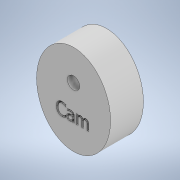
# Autodesk Inventor part: OVAAAAAL cam
Saved by Autodesk Inventor 2021 (Build 250183000, 183)
## iProperties
Created: 2021-04-14
Part Number: OVAAAAAL cam
Material: Generic
Document SubType Name: Modeling
Designer: Nabeel Azafer
Density: 1 g/cm^3
Appearance: Default
Author: Nabeel Azafer
Autodesk Inventor part; units mm, degrees
note: some values were not read from the file. Chosen so that the rebuilt part matches the saved one: direction of "Emboss1".
ref_plane "YZ Plane" through (0, 0, 0) normal (1, 0, 0) x (0, 1, 0)
ref_plane "XZ Plane" through (0, 0, 0) normal (0, 1, 0) x (-1, 0, 0)
ref_plane "XY Plane" through (0, 0, 0) normal (0, 0, 1) x (1, 0, 0)
sketch "Sketch1" plane through (0, 0, 0) normal (0, 0, 1) x (1, 0, 0)
  ellipse E0 centre (0, 0) end of major axis (0, 11) minor radius 9
  circle A0 centre (0, 3.5) radius 1.5
  dimension "d0" = 9
  dimension "d1" = 11
  dimension "d2" = 3
  dimension "d3" = 3.5
  constraints: 1 centre point, 1 coincident, 2 other
  measures "d2" diameter of A0
  measures "d3" distance of point (0, 0) A0.centre
extrude "Extrusion1" add sketch "Sketch1" along normal blind 8
sketch "Sketch2" plane through (0, 0, 8) normal (0, 0, 1) x (1, 0, 0)
  line L0 (-4.2953, -1.7977) -> (3.1049, -1.7977) construction
  line L1 (3.1049, -1.7977) -> (3.1049, -5.4978) construction
  line L2 (3.1049, -5.4978) -> (-4.2953, -5.4978) construction
  line L3 (-4.2953, -5.4978) -> (-4.2953, -1.7977) construction
  spline S0 degree 2 poles (-2.796, -4.9544) (-3.0924, -4.9544) (-3.5938, -4.7543) (-3.7766, -4.5542) knots 0 0 0 1 2 2 2
  spline S1 degree 2 poles (-3.7766, -4.5542) (-3.9594, -4.3566) (-4.1595, -3.7638) (-4.1595, -3.3785) knots 0 0 0 1 2 2 2
  spline S2 degree 2 poles (-4.1595, -3.3785) (-4.1595, -2.9956) (-3.9643, -2.4275) (-3.7791, -2.2176) knots 0 0 0 1 2 2 2
  spline S3 degree 2 poles (-3.7791, -2.2176) (-3.5963, -2.0126) (-3.0974, -1.7977) (-2.7886, -1.7977) knots 0 0 0 1 2 2 2
  spline S4 degree 2 poles (-2.7886, -1.7977) (-2.6355, -1.7977) (-2.3662, -1.8421) (-2.2526, -1.8767) knots 0 0 0 1 2 2 2
  spline S5 degree 2 poles (-2.2526, -1.8767) (-2.1538, -1.9088) (-1.9488, -2.0002) (-1.8475, -2.0546) knots 0 0 0 1 2 2 2
  line L4 (-1.8475, -2.0546) -> (-1.8475, -2.5436)
  line L5 (-1.8475, -2.5436) -> (-1.8796, -2.5436)
  spline S6 degree 2 poles (-1.8796, -2.5436) (-1.934, -2.4942) (-2.1019, -2.3559) (-2.223, -2.2892) knots 0 0 0 1 2 2 2
  spline S7 degree 2 poles (-2.223, -2.2892) (-2.3391, -2.225) (-2.6132, -2.1435) (-2.7911, -2.1435) knots 0 0 0 1 2 2 2
  spline S8 degree 2 poles (-2.7911, -2.1435) (-2.9862, -2.1435) (-3.3345, -2.304) (-3.4654, -2.4572) knots 0 0 0 1 2 2 2
  spline S9 degree 2 poles (-3.4654, -2.4572) (-3.5938, -2.6128) (-3.7371, -3.0846) (-3.7371, -3.3785) knots 0 0 0 1 2 2 2
  spline S10 degree 2 poles (-3.7371, -3.3785) (-3.7371, -3.6922) (-3.5864, -4.1442) (-3.4555, -4.2998) knots 0 0 0 1 2 2 2
  spline S11 degree 2 poles (-3.4555, -4.2998) (-3.3271, -4.4505) (-2.9837, -4.6036) (-2.7911, -4.6036) knots 0 0 0 1 2 2 2
  spline S12 degree 2 poles (-2.7911, -4.6036) (-2.6157, -4.6036) (-2.3168, -4.5172) (-2.2007, -4.4529) knots 0 0 0 1 2 2 2
  spline S13 degree 2 poles (-2.2007, -4.4529) (-2.0896, -4.3887) (-1.9241, -4.2553) (-1.8772, -4.2084) knots 0 0 0 1 2 2 2
  line L6 (-1.8772, -4.2084) -> (-1.8475, -4.2084)
  line L7 (-1.8475, -4.2084) -> (-1.8475, -4.6925)
  spline S14 degree 2 poles (-1.8475, -4.6925) (-1.9488, -4.7395) (-2.1266, -4.8259) (-2.2526, -4.8654) knots 0 0 0 1 2 2 2
  spline S15 degree 2 poles (-2.2526, -4.8654) (-2.386, -4.9099) (-2.6132, -4.9544) (-2.796, -4.9544) knots 0 0 0 1 2 2 2
  spline S16 degree 2 poles (-0.2247, -4.658) (-0.2717, -4.6925) (-0.4297, -4.816) (-0.5038, -4.8531) knots 0 0 0 1 2 2 2
  spline S17 degree 2 poles (-0.5038, -4.8531) (-0.6051, -4.9074) (-0.7953, -4.9642) (-0.9682, -4.9642) knots 0 0 0 1 2 2 2
  spline S18 degree 2 poles (-0.9682, -4.9642) (-1.109, -4.9642) (-1.3634, -4.858) (-1.4597, -4.7617) knots 0 0 0 1 2 2 2
  spline S19 degree 2 poles (-1.4597, -4.7617) (-1.5511, -4.6678) (-1.6623, -4.3912) (-1.6623, -4.2381) knots 0 0 0 1 2 2 2
  spline S20 degree 2 poles (-1.6623, -4.2381) (-1.6623, -4.0009) (-1.4622, -3.665) (-1.2449, -3.5687) knots 0 0 0 1 2 2 2
  spline S21 degree 2 poles (-1.2449, -3.5687) (-1.0522, -3.4798) (-0.5285, -3.4131) (-0.2247, -3.3958) knots 0 0 0 1 2 2 2
  line L8 (-0.2247, -3.3958) -> (-0.2247, -3.3217)
  spline S22 degree 2 poles (-0.2247, -3.3217) (-0.2247, -3.1883) (-0.3062, -3.0228) (-0.3803, -2.9759) knots 0 0 0 1 2 2 2
  spline S23 degree 2 poles (-0.3803, -2.9759) (-0.4544, -2.9289) (-0.6669, -2.8993) (-0.7805, -2.8993) knots 0 0 0 1 2 2 2
  spline S24 degree 2 poles (-0.7805, -2.8993) (-0.9139, -2.8993) (-1.2745, -2.9783) (-1.4548, -3.0549) knots 0 0 0 1 2 2 2
  line L9 (-1.4548, -3.0549) -> (-1.477, -3.0549)
  line L10 (-1.477, -3.0549) -> (-1.477, -2.6622)
  spline S25 degree 2 poles (-1.477, -2.6622) (-1.3708, -2.6325) (-0.9732, -2.5584) (-0.778, -2.5584) knots 0 0 0 1 2 2 2
  spline S26 degree 2 poles (-0.778, -2.5584) (-0.5409, -2.5584) (-0.2173, -2.6325) (-0.0889, -2.7289) knots 0 0 0 1 2 2 2
  spline S27 degree 2 poles (-0.0889, -2.7289) (0.0371, -2.8227) (0.1606, -3.1216) (0.1606, -3.3365) knots 0 0 0 1 2 2 2
  line L11 (0.1606, -3.3365) -> (0.1606, -4.9)
  line L12 (0.1606, -4.9) -> (-0.2247, -4.9)
  line L13 (-0.2247, -4.9) -> (-0.2247, -4.658)
  line L14 (-0.2247, -4.3369) -> (-0.2247, -3.7021)
  spline S28 degree 2 poles (-0.2247, -3.7021) (-0.3631, -3.7144) (-0.7805, -3.7564) (-0.9114, -3.7959) knots 0 0 0 1 2 2 2
  spline S29 degree 2 poles (-0.9114, -3.7959) (-1.0645, -3.8429) (-1.2646, -4.038) (-1.2646, -4.2109) knots 0 0 0 1 2 2 2
  spline S30 degree 2 poles (-1.2646, -4.2109) (-1.2646, -4.4085) (-1.0423, -4.6086) (-0.8299, -4.6086) knots 0 0 0 1 2 2 2
  spline S31 degree 2 poles (-0.8299, -4.6086) (-0.6496, -4.6086) (-0.3532, -4.4529) (-0.2247, -4.3369) knots 0 0 0 1 2 2 2
  line L15 (3.295, -4.9) -> (3.295, -3.5761)
  spline S32 degree 2 poles (3.295, -3.5761) (3.295, -3.418) (3.2703, -3.1488) (3.2308, -3.0747) knots 0 0 0 1 2 2 2
  spline S33 degree 2 poles (3.2308, -3.0747) (3.1913, -2.9932) (3.0406, -2.9141) (2.9097, -2.9141) knots 0 0 0 1 2 2 2
  spline S34 degree 2 poles (2.9097, -2.9141) (2.7912, -2.9141) (2.5195, -3.0599) (2.3762, -3.1982) knots 0 0 0 1 2 2 2
  spline S35 degree 2 poles (2.3762, -3.1982) (2.3787, -3.2328) (2.3836, -3.3291) (2.3836, -3.3933) knots 0 0 0 1 2 2 2
  line L16 (2.3836, -3.3933) -> (2.3836, -4.9)
  line L17 (2.3836, -4.9) -> (1.9983, -4.9)
  line L18 (1.9983, -4.9) -> (1.9983, -3.5761)
  spline S36 degree 2 poles (1.9983, -3.5761) (1.9983, -3.418) (1.9736, -3.1488) (1.9341, -3.0747) knots 0 0 0 1 2 2 2
  spline S37 degree 2 poles (1.9341, -3.0747) (1.8945, -2.9932) (1.7439, -2.9141) (1.613, -2.9141) knots 0 0 0 1 2 2 2
  spline S38 degree 2 poles (1.613, -2.9141) (1.4895, -2.9141) (1.2153, -3.0697) (1.0868, -3.1908) knots 0 0 0 1 2 2 2
  line L19 (1.0868, -3.1908) -> (1.0868, -4.9)
  line L20 (1.0868, -4.9) -> (0.7015, -4.9)
  line L21 (0.7015, -4.9) -> (0.7015, -2.6128)
  line L22 (0.7015, -2.6128) -> (1.0868, -2.6128)
  line L23 (1.0868, -2.6128) -> (1.0868, -2.8647)
  spline S39 degree 2 poles (1.0868, -2.8647) (1.2375, -2.7141) (1.5339, -2.5486) (1.7118, -2.5486) knots 0 0 0 1 2 2 2
  spline S40 degree 2 poles (1.7118, -2.5486) (1.9143, -2.5486) (2.228, -2.7338) (2.3095, -2.9438) knots 0 0 0 1 2 2 2
  spline S41 degree 2 poles (2.3095, -2.9438) (2.4849, -2.7486) (2.8159, -2.5486) (3.0085, -2.5486) knots 0 0 0 1 2 2 2
  spline S42 degree 2 poles (3.0085, -2.5486) (3.1567, -2.5486) (3.3988, -2.64) (3.4877, -2.7437) knots 0 0 0 1 2 2 2
  spline S43 degree 2 poles (3.4877, -2.7437) (3.5791, -2.8474) (3.6804, -3.1587) (3.6804, -3.3933) knots 0 0 0 1 2 2 2
  line L24 (3.6804, -3.3933) -> (3.6804, -4.9)
  line L25 (3.6804, -4.9) -> (3.295, -4.9)
  point P0 (0, 0)
  constraints: 2 other
emboss "Emboss1" sketch "Sketch2" operation cut depth 1 direction (0, 0, -1)
body "Solid1"
